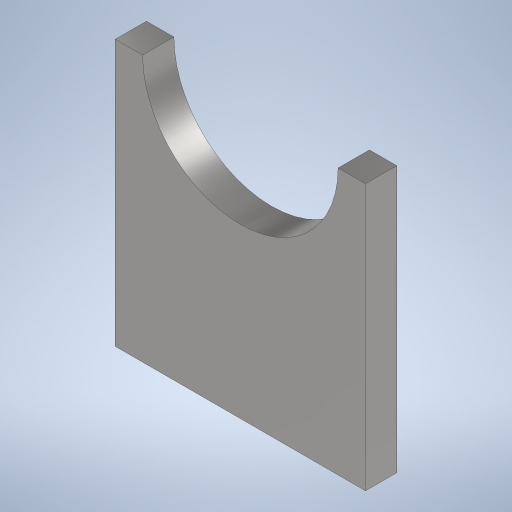
# Autodesk Inventor part: Weldedsupportpart1
Saved by Autodesk Inventor 2023 (Build 270158000, 158)
## iProperties
Created: 2022-09-04
Part Number: Weldedsupportpart1
Material: Steel, Mild
Document SubType Name: Modeling
Designer: Mike
Density: 7.85 g/cm^3
Appearance: Semi-Polished
Author: Mike
Autodesk Inventor part; units mm, degrees
ref_plane "YZ Plane" through (0, 0, 0) normal (1, 0, 0) x (0, 1, 0)
ref_plane "XZ Plane" through (0, 0, 0) normal (0, 1, 0) x (-1, 0, 0)
ref_plane "XY Plane" through (0, 0, 0) normal (0, 0, 1) x (1, 0, 0)
sketch "Sketch1" plane through (0, 0, 0) normal (0, 0, 1) x (1, 0, 0)
  line L0 (80, 170) -> (80, 0)
  line L1 (80, 0) -> (-80, 0)
  line L2 (-80, 0) -> (-80, 170)
  arc A0 (-62.5, 170) -> (62.5, 170) centre (0, 170) ccw
  line L3 (80, 170) -> (62.5, 170)
  line L4 (-80, 170) -> (-62.5, 170)
  point P0 (0, 0)
  point P1 (0, 0)
  point P2 (-71.25, 170)
  dimension "d9" = 80
  dimension "d10" = 80
  dimension "d12" = 160
  dimension "d14" = 125
  dimension "d15" = 170
  dimension "d16" = 170
  dimension "d17" = 17.5
  dimension "d18" = 17.5
  constraints: 10 end point, 2 horizontal, 2 midpoint, 2 perpendicular, 2 point on circle, 1 centre point, 1 vertical alignment
  measures "d9" distance of L1.end point (0, 0)
  measures "d10" distance of L0.end point (0, 0)
  measures "d12" distance between parallel lines of L0 L2
  measures "d14" diameter of A0
  measures "d15" distance of point (0, 0) A0.centre
  measures "d16" distance from line of point (-71.25, 170) L1
  measures "d17" distance of L4.end L2.end
  measures "d18" distance of L0.start L3.end
extrude "Extrusion1" add sketch "Sketch1" against normal blind 20
body "Solid1"
